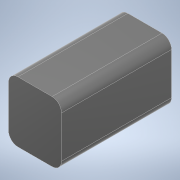
# Autodesk Inventor part: BH343
Saved by Autodesk Inventor 2022.2 (Build 262287010, 287A)
## iProperties
Created: 2024-06-30
Part Number: BH343
Material: 一般
Document SubType Name: Modeling
Designer: daisuke
Density: 1 g/cm^3
Appearance: 滑らか - 黒
Author: daisuke
Autodesk Inventor part; units mm, degrees
ref_plane "YZ Plane" through (0, 0, 0) normal (1, 0, 0) x (0, 1, 0)
ref_plane "XZ Plane" through (0, 0, 0) normal (0, 1, 0) x (-1, 0, 0)
ref_plane "XY Plane" through (0, 0, 0) normal (0, 0, 1) x (1, 0, 0)
sketch "スケッチ1" plane through (0, 0, 0) normal (0, 1, 0) x (-1, 0, 0)
  line L0 (14, -32) -> (-14, -32)
  line L1 (-14, -32) -> (-14, 0)
  line L2 (-14, 0) -> (14, 0)
  line L3 (14, 0) -> (14, -32)
  point P0 (0, 0)
  point P1 (0, 0)
  dimension "d0" = 28
  dimension "d1" = 32
  constraints: 8 end point, 2 parallel, 1 coincident, 1 horizontal, 1 midpoint, 1 perpendicular
  measures "d0" distance of L1.end L2.end
  measures "d1" distance of L0.end L1.end
extrude "押し出し1" add sketch "スケッチ1" along normal blind 58
fillet "フィレット1" radius 5 4 edges at (14, 29, 0) (-14, 29, 0) (14, 29, -32) (-14, 29, -32)
